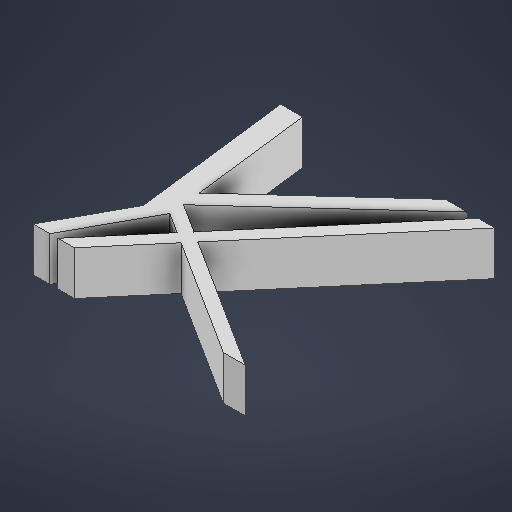
# Autodesk Inventor part: ESP32_C3_SM
Saved by Autodesk Inventor 2026.2 (Build 302298010, 298A)
## iProperties
Created: 2026-05-20
Part Number: ESP32_C3_SM
Material: Generic
Document SubType Name: Modeling
Designer: anton
Density: 1 g/cm^3
Appearance: Default
Author: anton
Autodesk Inventor part; units mm, degrees
ref_plane "YZ Plane" through (0, 0, 0) normal (1, 0, 0) x (0, 1, 0)
ref_plane "XZ Plane" through (0, 0, 0) normal (0, 1, 0) x (-1, 0, 0)
ref_plane "XY Plane" through (0, 0, 0) normal (0, 0, 1) x (1, 0, 0)
sketch "Sketch1" plane through (0, 0, 0) normal (0, 1, 0) x (-1, 0, 0)
  line L0 (22.5, 0) -> (22.5, -17.7)
  line L1 (0, -17.7) -> (0, 0)
  line L2 (0, -17.7) -> (0, -18.7)
  line L3 (22.5, -18.7) -> (22.5, -17.7)
  line L4 (22.5, -18.7) -> (22.5, -20.7)
  line L5 (22.5, -20.7) -> (0, -20.7)
  line L6 (0, -20.7) -> (0, -18.7)
  line L7 (22.5, -5.2144) -> (27.7427, -5.2144)
  line L8 (27.7427, -5.2144) -> (27.7427, -12.0619)
  line L9 (27.7427, -12.0619) -> (22.5, -12.0619)
  line L10 (22.5, -12.0619) -> (22.5, -5.2144)
  line L11 (22.5, -18.7) -> (20.5, -18.7)
  line L12 (20.5, -18.7) -> (20.5, -20.7)
  line L13 (20.5, -20.7) -> (22.5, -20.7)
  line L14 (22.5, -20.7) -> (22.5, -18.7)
  line L15 (20.5, -20.7) -> (19.5, -20.7)
  line L16 (19.5, -20.7) -> (19.5, -18.7)
  line L17 (19.5, -18.7) -> (20.5, -18.7)
  line L18 (20.5, -18.7) -> (20.5, -20.7)
  line L19 (19.5, -20.7) -> (17.8475, -7.1514)
  line L20 (2.5, -20.7) -> (15.9946, -8.3576)
  line L21 (4.5, -20.7) -> (16.1953, -10.0032)
  line L22 (19.7898, 0) -> (15.8518, -7.1866)
  line L23 (21.3117, 0) -> (17.7647, -6.4729)
  line L24 (17.7647, -6.4729) -> (17.8475, -7.1514)
  line L25 (2.546, 1.4707) -> (0.546, 1.4707)
  line L26 (17.5, -20.7) -> (16.1953, -10.0032)
  line L27 (15.8518, -7.1866) -> (15.8475, -7.1514)
  line L28 (1.5, -20.7) -> (13.3825, -6.6958)
  line L29 (14.0836, -5.8694) -> (19.0638, 0)
  line L30 (0, -20.7) -> (12.4083, -6.076)
  line L31 (13.1095, -5.2497) -> (17.5638, 0)
  line L32 (15.9946, -8.3576) -> (13.3825, -6.6958)
  line L33 (12.4083, -6.076) -> (0.546, 1.4707)
  line L34 (15.9299, -7.044) -> (14.0836, -5.8694)
  line L35 (13.1095, -5.2497) -> (2.546, 1.4707)
  line L36 (0, 0) -> (2.8578, 0)
  line L37 (4.8578, 0) -> (22.5, 0)
  line L38 (19.2561, -18.7) -> (22.5, -18.7)
  line L39 (19.2561, -18.7) -> (22.5, -18.7)
  line L40 (22.5, -17.7) -> (19.1341, -17.7)
  line L41 (22.5, -17.7) -> (19.1341, -17.7)
  line L42 (6.6867, -18.7) -> (17.2561, -18.7)
  line L43 (6.6867, -18.7) -> (17.2561, -18.7)
  line L44 (17.1341, -17.7) -> (7.7801, -17.7)
  line L45 (17.1341, -17.7) -> (7.7801, -17.7)
  line L46 (0, -18.7) -> (1.697, -18.7)
  line L47 (3.197, -18.7) -> (4.6867, -18.7)
  line L48 (0, -18.7) -> (1.697, -18.7)
  line L49 (3.197, -18.7) -> (4.6867, -18.7)
  line L50 (5.7801, -17.7) -> (4.0455, -17.7)
  line L51 (2.5455, -17.7) -> (0, -17.7)
  line L52 (5.7801, -17.7) -> (4.0455, -17.7)
  line L53 (2.5455, -17.7) -> (0, -17.7)
  point P0 (0, -8.85)
  dimension "d0" = 22.5
  dimension "d1" = 17.7
  dimension "d10" = 2
  dimension "d11" = 2
  dimension "d12" = 1
  constraints: 108 end point, 49 parallel, 24 point on line, 14 horizontal, 13 perpendicular, 1 midpoint
  measures "d0" distance of L0.end L1.start
  measures "d1" distance of L0.start L0.end
  measures "d10" distance of L4.start L4.end
  measures "d11" distance of L13.end L12.end
  measures "d12" distance of L16.end L17.end
extrude "Extrusion3" add sketch "Sketch1" along normal blind 4 contours L23 L24 L19 L5 L26 L21 L20 L32 L28 L30 L33 L25 L35 L31 L37 L29 L34 L22
body "Solid3"
